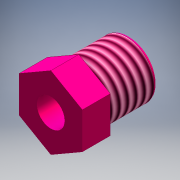
# Autodesk Inventor part: Premistoppa M10x1
Saved by Autodesk Inventor 2016 (Build 200138000, 138)
## iProperties
Created: 2016-09-10
Part Number: Premistoppa M10x1
Material: Generic
Document SubType Name: Modeling
Designer: Muhammad
Density: 1 g/cm^3
Appearance: Default
Author: Muhammad
Autodesk Inventor part; units mm, degrees
ref_plane "YZ Plane" through (0, 0, 0) normal (1, 0, 0) x (0, 1, 0)
ref_plane "XZ Plane" through (0, 0, 0) normal (0, 1, 0) x (-1, 0, 0)
ref_plane "XY Plane" through (0, 0, 0) normal (0, 0, 1) x (1, 0, 0)
sketch "Sketch1" plane through (0, 0, 0) normal (0, 1, 0) x (-1, 0, 0)
  line L0 (0, 0) -> (0, -6.5) construction
  line L1 (0, -6.5) -> (0, 6.5) construction
  line L2 (0, -6.5) -> (-5.6292, -3.25)
  line L3 (-5.6292, -3.25) -> (-5.6292, 3.25)
  line L4 (-5.6292, 3.25) -> (0, 6.5)
  line L5 (0, 6.5) -> (5.6292, 3.25)
  line L6 (5.6292, 3.25) -> (5.6292, -3.25)
  line L7 (5.6292, -3.25) -> (0, -6.5)
  constraints: 16 end point, 1 coincident, 1 point on line, 1 vertical, 13 other
extrude "Extrusion1" add sketch "Sketch1" along normal blind 5
sketch "Sketch2" plane through (0, 5, 0) normal (0, 1, 0) x (1, 0, 0)
  circle A0 centre (0, 0) radius 2.5
  circle A1 centre (0, 0) radius 5
  dimension "d4" = 5
  dimension "d5" = 10
  constraints: 2 centre point, 2 coincident
  measures "d4" diameter of A0
  measures "d5" diameter of A1
extrude "Extrusion2" add sketch "Sketch2" along normal blind 9
sketch "Sketch3" plane through (0, 5, 0) normal (0, 1, 0) x (1, 0, 0)
  circle A0 centre (0, 0) radius 2.5
  constraints: 1 centre point, 1 coincident
extrude "Extrusion3" cut sketch "Sketch3" against normal through all
thread "Thread1" size "M10x1.5" class "6g" standard "ANSI Metric M Profile" full length
fillet "Fillet1" radius 0.5 1 edges at (-5, 14, 0)
body "Solid1"
